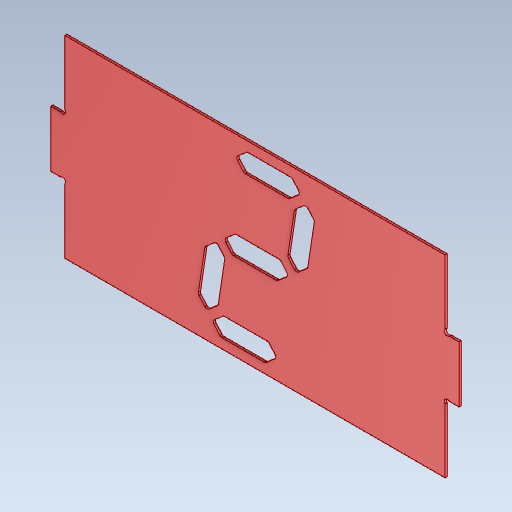
# Autodesk Inventor part: Cockpit_front_frame_cloth
Saved by Autodesk Inventor 2020 (Build 240168000, 168)
## iProperties
Part Number: Cockpit_front_frame_cloth
Material: PET プラスチック
Document SubType Name: Modeling
Designer: Masato Kubotera
Density: 1.541 g/cm^3
Appearance: 滑らか - 赤
Description: PP T0.75
Mass: 10.1319 g
Surface Area: 180.446 cm^2
Volume: 6.57488 cm^3
Author: Masato Kubotera
Autodesk Inventor part; units mm, degrees
ref_plane "YZ Plane" through (0, 0, 0) normal (1, 0, 0) x (0, 1, 0)
ref_plane "XZ Plane" through (0, 0, 0) normal (0, 1, 0) x (-1, 0, 0)
ref_plane "XY Plane" through (0, 0, 0) normal (0, 0, 1) x (1, 0, 0)
derived "Cockpit_front_frame.ipt"
sketch "スケッチ2" plane through (0, 0, 0) normal (0, 1, 0) x (-1, 0, 0)
  line L0 (-23.5, -22.5) -> (-28.5, -27.5)
  line L1 (-28.5, -27.5) -> (-28.5, -91)
  line L2 (-28.5, -91) -> (-23.5, -96)
  line L3 (-23.5, -96) -> (34.25, -96)
  line L4 (36.25, -98) -> (36.25, -131)
  line L5 (36.25, -131) -> (41.25, -136)
  line L6 (41.25, -136) -> (86.5, -136)
  line L7 (91.5, -131) -> (91.5, -20)
  line L8 (91.5, -20) -> (89, -17.5)
  line L9 (89, -17.5) -> (83.25, -17.5)
  line L10 (83.25, -17.5) -> (83.25, -21.0151)
  line L11 (81.7651, -22.5) -> (76.9849, -22.5)
  line L12 (75.5, -21.0151) -> (75.5, -17.5)
  line L13 (75.5, -17.5) -> (67.5, -17.5)
  line L14 (67.5, -17.5) -> (67.5, -21.0151)
  line L15 (66.0151, -22.5) -> (-23.5, -22.5)
  line L16 (-25.25, -25) -> (-20.25, -25) construction
  line L17 (-20.25, -25) -> (-20.25, -93.5) construction
  line L18 (-20.25, -93.5) -> (-25.25, -93.5) construction
  line L19 (-25.25, -93.5) -> (-25.25, -25) construction
  line L20 (-26, -25) -> (-25.25, -25) construction
  line L21 (-25.25, -93.5) -> (-26, -93.5) construction
  line L22 (-26, -93.5) -> (-26, -25) construction
  line L23 (-20.25, -93.5) -> (83.25, -93.5) construction
  line L24 (-20.25, -88.5) -> (83.25, -88.5) construction
  line L25 (83.25, -22.5) -> (83.25, -90.5) construction
  line L26 (83.25, -90.5) -> (88.25, -90.5) construction
  line L27 (88.25, -90.5) -> (88.25, -22.5) construction
  line L28 (83.25, -88.5) -> (83.25, -93.5) construction
  line L29 (83.25, -91) -> (88.25, -91) construction
  line L30 (88.25, -91) -> (88.25, -133.5) construction
  line L31 (83.25, -91) -> (83.25, -133.5) construction
  line L32 (83.25, -133.5) -> (88.25, -133.5) construction
  line L33 (38.75, -133.5) -> (38.75, -128.5) construction
  line L34 (38.75, -128.5) -> (38.75, -93.5) construction
  line L35 (43.75, -93.5) -> (43.75, -128.5) construction
  line L36 (38.75, -128.5) -> (43.75, -128.5) construction
  line L37 (41.25, -128.5) -> (41.25, -93.5) construction
  line L38 (38.75, -128.5) -> (82.1145, -128.5) construction
  line L39 (82.1145, -128.5) -> (82.1145, -133.5) construction
  line L40 (82.1145, -133.5) -> (38.75, -133.5) construction
  line L41 (38.75, -131) -> (82.1145, -131) construction
  line L42 (85.75, -91) -> (85.75, -133.5) construction
  circle A0 centre (85.75, -131) radius 2
  arc A1 (83.25, -128.5) -> (88.25, -128.5) centre (85.75, -131) ccw construction
  line L43 (83.25, -91) -> (-20.25, -91) construction
  line L44 (41.25, -111) -> (43.75, -111) construction
  line L45 (60.4322, -128.5) -> (60.4322, -131) construction
  line L46 (41.2, -115.5651) -> (41.2, -106.4349)
  line L47 (43.8, -107.05) -> (43.8, -114.95)
  line L48 (43.8, -117.05) -> (41.2, -104.95) construction
  line L49 (41.2, -117.05) -> (43.8, -104.95) construction
  line L50 (56.4822, -128.45) -> (64.3822, -128.45)
  line L51 (64.9973, -131.05) -> (55.8672, -131.05)
  line L52 (54.3822, -128.45) -> (66.4822, -131.05) construction
  line L53 (66.4822, -128.45) -> (54.3822, -131.05) construction
  line L54 (41.25, -105) -> (43.75, -105) construction
  line L55 (41.25, -117) -> (43.75, -117) construction
  arc A2 (42.6849, -104.95) -> (41.2, -106.4349) centre (41.9425, -105.6925) ccw
  arc A3 (43.8, -107.05) -> (43.8, -104.95) centre (43.8, -106) ccw
  arc A4 (41.2, -115.5651) -> (42.6849, -117.05) centre (41.9425, -116.3075) ccw
  arc A5 (43.8, -117.05) -> (43.8, -114.95) centre (43.8, -116) ccw
  line L56 (54.4322, -131) -> (54.4322, -128.5) construction
  line L57 (66.4322, -128.5) -> (66.4322, -131) construction
  arc A6 (54.3822, -129.5651) -> (55.8672, -131.05) centre (55.1247, -130.3075) ccw
  arc A7 (56.4822, -128.45) -> (54.3822, -128.45) centre (55.4322, -128.45) ccw
  arc A8 (64.9973, -131.05) -> (66.4822, -129.5651) centre (65.7398, -130.3075) ccw
  arc A9 (66.4822, -128.45) -> (64.3822, -128.45) centre (65.4322, -128.45) ccw
  line L58 (54.3822, -129.5651) -> (54.3822, -128.45)
  line L59 (66.4822, -128.45) -> (66.4822, -129.5651)
  line L60 (42.6849, -104.95) -> (43.8, -104.95)
  line L61 (43.8, -117.05) -> (42.6849, -117.05)
  circle A10 centre (48.4322, -131) radius 1.6
  line L62 (88.25, -22.5) -> (88.25, -17.5) construction
  line L63 (89, -17.5) -> (89, -90.5) construction
  line L64 (89, -90.5) -> (88.25, -90.5) construction
  line L65 (-13.5, -82.5) -> (-13.5, -61)
  arc A11 (-13.5, -82.5) -> (-11.5, -84.5) centre (-11.5, -82.5) ccw
  line L66 (45.5, -84.5) -> (-11.5, -84.5)
  arc A12 (45.5, -84.5) -> (47.5, -82.5) centre (45.5, -82.5) ccw
  line L67 (47.5, -61) -> (47.5, -82.5)
  arc A13 (47.5, -61) -> (45.5, -59) centre (45.5, -61) ccw
  line L68 (-11.5, -59) -> (45.5, -59)
  arc A14 (-11.5, -59) -> (-13.5, -61) centre (-11.5, -61) ccw
  line L69 (31.5, -88.5) -> (31.5, -91) construction
  line L70 (85.75, -22.5) -> (85.75, -90.5) construction
  circle A15 centre (85.75, -34) radius 1.6
  circle A16 centre (85.75, -34) radius 3
  circle A17 centre (85.75, -79) radius 1.6
  circle A18 centre (85.75, -79) radius 3
  line L71 (88.25, -22.5) -> (83.25, -22.5) construction
  arc A19 (88.25, -91) -> (83.25, -91) centre (85.75, -131) ccw construction
  circle A20 centre (48.4322, -131) radius 3
  circle A21 centre (41.25, -99) radius 1.6
  circle A22 centre (41.25, -99) radius 3
  line L72 (6.5, -88.5) -> (6.5, -91) construction
  line L73 (56.5, -88.5) -> (56.5, -91) construction
  line L74 (55.0651, -91.05) -> (7.9349, -91.05)
  line L75 (6.45, -89.5651) -> (6.45, -88.45)
  line L76 (8.55, -88.45) -> (54.45, -88.45)
  line L77 (56.55, -88.45) -> (56.55, -89.5651)
  line L78 (56.55, -91.05) -> (6.45, -88.45) construction
  line L79 (6.45, -91.05) -> (56.55, -88.45) construction
  arc A23 (8.55, -88.45) -> (6.45, -88.45) centre (7.5, -88.45) ccw
  arc A24 (6.45, -89.5651) -> (7.9349, -91.05) centre (7.1925, -90.3075) ccw
  arc A25 (56.55, -88.45) -> (54.45, -88.45) centre (55.5, -88.45) ccw
  arc A26 (55.0651, -91.05) -> (56.55, -89.5651) centre (55.8075, -90.3075) ccw
  line L80 (-20.25, -41) -> (83.25, -41) construction
  line L81 (83.25, -36) -> (-20.25, -36) construction
  line L82 (-20.25, -36) -> (-20.25, -41) construction
  line L83 (-20.25, -38.5) -> (83.25, -38.5) construction
  line L84 (31.5, -41) -> (31.5, -36) construction
  line L85 (55.0651, -35.95) -> (7.9349, -35.95)
  line L86 (7.9349, -41.05) -> (55.0651, -41.05)
  line L87 (56.55, -35.95) -> (6.45, -41.05) construction
  line L88 (6.45, -35.95) -> (55.5877, -40.952) construction
  arc A27 (7.9349, -35.95) -> (6.45, -37.4349) centre (7.1925, -36.6925) ccw
  arc A28 (6.45, -39.5651) -> (7.9349, -41.05) centre (7.1925, -40.3075) ccw
  arc A29 (56.55, -37.4349) -> (55.0651, -35.95) centre (55.8075, -36.6925) ccw
  arc A30 (55.0651, -41.05) -> (56.55, -39.5651) centre (55.8075, -40.3075) ccw
  line L89 (6.5, -41) -> (6.5, -36) construction
  line L90 (56.5, -36) -> (56.5, -41) construction
  line L91 (6.45, -37.4349) -> (6.45, -39.5651)
  line L92 (56.55, -39.5651) -> (56.55, -37.4349)
  circle A31 centre (-1, -38.5) radius 1.6
  circle A32 centre (-1, -38.5) radius 3
  circle A33 centre (64, -38.5) radius 1.6
  circle A34 centre (64, -38.5) radius 3
  line L93 (-25.25, -49.25) -> (-26, -49.25) construction
  line L94 (-25.25, -69.25) -> (-26, -69.25) construction
  line L95 (-26, -59.25) -> (-25.25, -59.25) construction
  line L96 (-22.75, -25) -> (-22.75, -93.5) construction
  arc A35 (66.0151, -22.5) -> (67.5, -21.0151) centre (66.7575, -21.7575) ccw
  arc A36 (75.5, -21.0151) -> (76.9849, -22.5) centre (76.2425, -21.7575) ccw
  line L97 (59.75, -22.5) -> (59.75, -32.5) construction
  line L98 (59.75, -32.5) -> (83.25, -32.5) construction
  line L99 (83.25, -32.5) -> (83.25, -22.5) construction
  line L100 (71.5, -17.5) -> (71.5, -32.5) construction
  line L101 (63.5, -22.5) -> (63.5, -17.5) construction
  line L102 (79.5, -22.5) -> (79.5, -17.5) construction
  circle A37 centre (-22.75, -31.75) radius 1.6
  circle A38 centre (-22.75, -31.75) radius 3
  circle A39 centre (-22.75, -86.75) radius 1.6
  circle A40 centre (-22.75, -86.75) radius 3
  line L103 (67.5, -22.5) -> (75.5, -22.5)
  line L104 (88.25, -17.5) -> (52.5, -17.5) construction
  line L105 (52.5, -17.5) -> (52.5, -22.5) construction
  circle A41 centre (85.75, -98.5) radius 1.475
  circle A42 centre (85.75, -103.5) radius 1.475
  circle A43 centre (85.75, -108.5) radius 1.475
  line L106 (48.25, -93.5) -> (78.75, -93.5)
  line L107 (80.75, -95.5) -> (80.75, -124)
  line L108 (78.75, -126) -> (48.25, -126)
  line L109 (46.25, -124) -> (46.25, -95.5)
  arc A44 (48.25, -93.5) -> (46.25, -95.5) centre (48.25, -95.5) ccw
  arc A45 (46.25, -124) -> (48.25, -126) centre (48.25, -124) ccw
  arc A46 (78.75, -126) -> (80.75, -124) centre (78.75, -124) ccw
  arc A47 (80.75, -95.5) -> (78.75, -93.5) centre (78.75, -95.5) ccw
  arc A48 (36.25, -98) -> (34.25, -96) centre (34.25, -98) ccw
  circle A49 centre (-13.5, -55) radius 1.75
  circle A50 centre (-13.5, -55) radius 2
  line L110 (77.85, -78.65) -> (68.65, -78.65) construction
  line L111 (68.65, -78.65) -> (68.65, -64.85) construction
  line L112 (68.65, -64.85) -> (77.85, -64.85) construction
  line L113 (77.85, -64.85) -> (77.85, -78.65) construction
  line L114 (77.85, -78.65) -> (68.65, -64.85) construction
  line L115 (68.65, -78.65) -> (77.85, -64.85) construction
  line L116 (67.95, -64.2) -> (78.55, -64.2) construction
  line L117 (78.55, -64.2) -> (78.55, -79.3) construction
  line L118 (78.55, -79.3) -> (67.95, -79.3) construction
  line L119 (67.95, -79.3) -> (67.95, -64.2) construction
  line L120 (67.95, -64.2) -> (78.55, -79.3) construction
  line L121 (78.55, -64.2) -> (67.95, -79.3) construction
  line L122 (69.3849, -64.15) -> (77.1151, -64.15)
  line L123 (78.6, -65.6349) -> (78.6, -77.8651)
  line L124 (78.6, -79.35) -> (67.9, -64.15) construction
  line L125 (67.9, -79.35) -> (78.6, -64.15) construction
  line L126 (77.9, -78.7) -> (68.6, -64.8) construction
  line L127 (68.6, -78.7) -> (77.9, -64.8) construction
  arc A51 (69.3849, -64.15) -> (67.9, -65.6349) centre (68.6425, -64.8925) ccw
  arc A52 (70.0849, -64.8) -> (68.6, -66.2849) centre (69.3425, -65.5425) ccw
  line L128 (67.9, -71.75) -> (78.6, -71.75) construction
  line L129 (73.25, -64.15) -> (73.25, -78.7063) construction
  arc A53 (78.6, -65.6349) -> (77.1151, -64.15) centre (77.8575, -64.8925) ccw
  arc A54 (77.9, -66.2849) -> (76.4151, -64.8) centre (77.1575, -65.5425) ccw
  arc A55 (67.9, -77.8651) -> (69.3849, -79.35) centre (68.6425, -78.6075) ccw
  arc A56 (68.6, -77.2151) -> (70.0849, -78.7) centre (69.3425, -77.9575) ccw
  arc A57 (77.1151, -79.35) -> (78.6, -77.8651) centre (77.8575, -78.6075) ccw
  arc A58 (76.4151, -78.7) -> (77.9, -77.2151) centre (77.1575, -77.9575) ccw
  line L130 (70.0849, -64.8) -> (76.4151, -64.8)
  line L131 (77.9, -66.2849) -> (77.9, -77.2151)
  line L132 (67.9, -77.8651) -> (67.9, -65.6349)
  line L133 (68.6, -77.2151) -> (68.6, -66.2849)
  line L134 (76.4151, -78.7) -> (70.0849, -78.7)
  line L135 (77.1151, -79.35) -> (69.3849, -79.35)
  line L136 (-13.5, -71.75) -> (47.5, -71.75) construction
  line L137 (85.75, -56.5) -> (88.25, -56.5) construction
  line L138 (89, -54) -> (88.25, -54) construction
  line L139 (85.7, -69.45) -> (85.7, -43.55)
  line L140 (88.2835, -71.3588) -> (85.7, -41.45) construction
  line L141 (85.7, -71.55) -> (88.3, -41.45) construction
  arc A59 (85.7, -41.45) -> (85.7, -43.55) centre (85.7, -42.5) ccw
  arc A60 (88.3, -42.9349) -> (86.8151, -41.45) centre (87.5575, -42.1925) ccw
  arc A61 (85.7, -69.45) -> (85.7, -71.55) centre (85.7, -70.5) ccw
  arc A62 (86.8151, -71.55) -> (88.3, -70.0651) centre (87.5575, -70.8075) ccw
  line L142 (85.75, -41.5) -> (88.25, -41.5) construction
  line L143 (85.75, -71.5) -> (88.25, -71.5) construction
  arc A63 (89.25, -47.1801) -> (88.3, -46.1348) centre (88.2, -47.1801) ccw
  line L144 (89.25, -47.1801) -> (89.25, -65.8199)
  line L145 (88.25, -46.5) -> (89, -46.5) construction
  line L146 (88.25, -66.5) -> (89, -66.5) construction
  arc A64 (88.3, -66.8652) -> (89.25, -65.8199) centre (88.2, -65.8199) ccw
  line L147 (88.3, -42.9349) -> (88.3, -46.1348)
  line L148 (88.3, -66.8652) -> (88.3, -70.0651)
  line L149 (86.8151, -71.55) -> (85.7, -71.55)
  line L150 (85.7, -41.45) -> (86.8151, -41.45)
  line L151 (86.5, -136) -> (91.5, -131)
  arc A65 (81.7651, -22.5) -> (83.25, -21.0151) centre (82.5075, -21.7575) ccw
  circle A66 centre (85.75, -93.5) radius 2
  circle A67 centre (85.75, -93.5) radius 4 construction
  arc A68 (-24.15, -49.25) -> (-26.25, -49.25) centre (-25.2, -49.25) ccw
  line L152 (-26, -49.25) -> (-26.25, -49.25) construction
  line L153 (-26.25, -49.25) -> (-26.25, -69.25)
  line L154 (-24.15, -49.25) -> (-24.15, -69.25)
  arc A69 (-26.25, -69.25) -> (-24.15, -69.25) centre (-25.2, -69.25) ccw
  point P0 (0, 0)
  point P1 (-25.7227, -96)
  point P2 (-23.5, -22.5)
  point P3 (42.5, -111)
  point P4 (60.4322, -129.75)
  point P5 (31.5, -89.75)
  point P6 (31.5, -38.5)
  point P7 (6.45, -41.05)
  point P8 (52.5, -22)
  point P9 (73.25, -71.75)
  point P10 (73.25, -71.75)
  point P11 (87, -56.5)
  dimension "d4" = 0.75
  measures "d4" distance of L20.start L20.end
sketch "スケッチ3" plane through (25.25, 0, 0) normal (1, 0, 0) x (0, 1, 0)
  line L0 (-135, -25) -> (0, -25)
  line L1 (0, -93.5) -> (-135, -93.5)
  line L2 (0, -25) -> (0, -93.5)
  line L3 (0, -75.7349) -> (0, -93.5)
  line L4 (-67.5, -25) -> (-67.5, -93.5) construction
  line L5 (-135, -25) -> (-135, -93.5)
  line L6 (-7, -30) -> (-128, -30)
  line L7 (-130, -32) -> (-130, -34)
  line L8 (-128, -36) -> (-7, -36)
  line L9 (-5, -34) -> (-5, -32)
  line L10 (-5, -30) -> (-130, -36) construction
  line L11 (-130, -30) -> (-5, -36) construction
  line L12 (-7, -88.5) -> (-128, -88.5)
  line L13 (-130, -86.5) -> (-130, -43)
  line L14 (-128, -41) -> (-7, -41)
  line L15 (-5, -43) -> (-5, -86.5)
  line L16 (-5, -88.5) -> (-130, -41) construction
  line L17 (-130, -88.5) -> (-5, -41) construction
  arc A0 (-128, -30) -> (-130, -32) centre (-128, -32) ccw
  arc A1 (-130, -34) -> (-128, -36) centre (-128, -34) ccw
  arc A2 (-7, -36) -> (-5, -34) centre (-7, -34) ccw
  arc A3 (-5, -32) -> (-7, -30) centre (-7, -32) ccw
  arc A4 (-5, -43) -> (-7, -41) centre (-7, -43) ccw
  arc A5 (-128, -41) -> (-130, -43) centre (-128, -43) ccw
  arc A6 (-130, -86.5) -> (-128, -88.5) centre (-128, -86.5) ccw
  arc A7 (-7, -88.5) -> (-5, -86.5) centre (-7, -86.5) ccw
  point P0 (0, 0)
  point P1 (-135, -93.5)
  point P2 (-135, -25)
  point P3 (-67.5, -33)
  point P4 (-67.5, -64.75)
  point P5 (0, -36)
  point P6 (0, -36)
  point P7 (0, -36)
  point P8 (0, -41)
  point P9 (0, -41)
  point P10 (0, -41)
ref_plane "作業平面1" through (25.25, -135, -25) normal (-1, 0, 0) x (0, 1, 0)
sketch "スケッチ4" plane through (25.25, -135, -25) normal (-1, 0, 0) x (0, 1, 0)
  arc A0 (136.4849, 24.25) -> (135, 22.7651) centre (135.7425, 23.5075) ccw
  line L0 (136.4849, 24.25) -> (140, 24.25)
  line L1 (140, 24.25) -> (140, 44.25)
  line L2 (67.5, 0) -> (67.5, 68.5) construction
  line L3 (0, 0) -> (135, 0) projected
  line L4 (135, 68.5) -> (0, 68.5) projected
  arc A1 (135, 45.7349) -> (136.4849, 44.25) centre (135.7425, 44.9925) ccw
  line L5 (136.4849, 44.25) -> (140, 44.25)
  line L6 (135, 22.7651) -> (135, 0)
  line L7 (135, 45.7349) -> (135, 68.5)
  arc A2 (0, 22.7651) -> (-1.4849, 24.25) centre (-0.7425, 23.5075) ccw
  line L8 (-1.4849, 24.25) -> (-5, 24.25)
  line L9 (-1.4849, 44.25) -> (-5, 44.25)
  arc A3 (-1.4849, 44.25) -> (0, 45.7349) centre (-0.7425, 44.9925) ccw
  line L10 (0, 22.7651) -> (0, 0)
  line L11 (0, 45.7349) -> (0, 68.5)
  line L12 (-5, 24.25) -> (-5, 44.25)
  line L13 (51.1141, 58.6095) -> (54.1517, 56.0021)
  line L14 (53.0682, 60.8859) -> (56.1057, 58.2784)
  line L15 (55.0145, 64.6885) -> (52.9607, 62.296)
  line L16 (49.704, 58.5021) -> (47.6502, 56.1095)
  line L17 (55.7733, 65.0372) -> (70.8617, 65.0372)
  line L18 (72.6043, 58.3859) -> (74.658, 60.7784)
  line L19 (71.513, 64.796) -> (74.5506, 62.1885)
  line L20 (56.7571, 58.0372) -> (71.8455, 58.0372)
  line L21 (54.4888, 55.3948) -> (56.7748, 40.4805)
  line L22 (56.5452, 39.6777) -> (54.4914, 37.2851)
  line L23 (53.0813, 37.1777) -> (50.0437, 39.7851)
  line L24 (47.4206, 55.3066) -> (49.7066, 40.3924)
  line L25 (50.3553, 59.2608) -> (53.84, 36.5264) construction
  line L26 (75.3094, 61.5372) -> (52.3094, 61.5372) construction
  arc A4 (51.1141, 58.6095) -> (49.704, 58.5021) centre (50.4628, 57.8507) ccw
  arc A5 (54.4888, 55.3948) -> (54.1517, 56.0021) centre (53.5003, 55.2433) ccw
  arc A6 (56.5452, 39.6777) -> (56.7748, 40.4805) centre (55.7864, 40.329) ccw
  arc A7 (53.0813, 37.1777) -> (54.4914, 37.2851) centre (53.7326, 37.9365) ccw
  arc A8 (49.7066, 40.3924) -> (50.0437, 39.7851) centre (50.695, 40.5439) ccw
  arc A9 (47.6502, 56.1095) -> (47.4206, 55.3066) centre (48.409, 55.4582) ccw
  arc A10 (71.8455, 58.0372) -> (72.6043, 58.3859) centre (71.8455, 59.0372) ccw
  arc A11 (74.658, 60.7784) -> (74.5506, 62.1885) centre (73.8992, 61.4298) ccw
  arc A12 (71.513, 64.796) -> (70.8617, 65.0372) centre (70.8617, 64.0372) ccw
  arc A13 (55.7733, 65.0372) -> (55.0145, 64.6885) centre (55.7733, 64.0372) ccw
  arc A14 (52.9607, 62.296) -> (53.0682, 60.8859) centre (53.7195, 61.6446) ccw
  arc A15 (56.1057, 58.2784) -> (56.7571, 58.0372) centre (56.7571, 59.0372) ccw
  line L27 (78.72, 58.6095) -> (81.7576, 56.0021)
  line L28 (77.3099, 58.5021) -> (75.2561, 56.1095)
  arc A16 (78.72, 58.6095) -> (77.3099, 58.5021) centre (78.0687, 57.8507) ccw
  line L29 (75.0264, 55.3066) -> (77.3125, 40.3924)
  arc A17 (75.2561, 56.1095) -> (75.0264, 55.3066) centre (76.0149, 55.4582) ccw
  arc A18 (82.0947, 55.3948) -> (81.7576, 56.0021) centre (81.1062, 55.2433) ccw
  line L30 (82.0947, 55.3948) -> (84.3807, 40.4805)
  arc A19 (84.151, 39.6777) -> (84.3807, 40.4805) centre (83.3922, 40.329) ccw
  line L31 (84.151, 39.6777) -> (82.0973, 37.2851)
  arc A20 (80.6871, 37.1777) -> (82.0973, 37.2851) centre (81.3385, 37.9365) ccw
  line L32 (80.6871, 37.1777) -> (77.6496, 39.7851)
  arc A21 (77.3125, 40.3924) -> (77.6496, 39.7851) centre (78.3009, 40.5439) ccw
  line L33 (55.2967, 31.3223) -> (58.3342, 28.7149)
  line L34 (53.8865, 31.2149) -> (51.8328, 28.8223)
  arc A22 (55.2967, 31.3223) -> (53.8865, 31.2149) centre (54.6453, 30.5635) ccw
  line L35 (51.6031, 28.0195) -> (53.8891, 13.1052)
  arc A23 (51.8328, 28.8223) -> (51.6031, 28.0195) centre (52.5915, 28.171) ccw
  arc A24 (58.6713, 28.1076) -> (58.3342, 28.7149) centre (57.6829, 27.9561) ccw
  line L36 (58.6713, 28.1076) -> (60.9573, 13.1934)
  arc A25 (60.7277, 12.3905) -> (60.9573, 13.1934) centre (59.9689, 13.0418) ccw
  line L37 (60.7277, 12.3905) -> (58.6739, 9.9979)
  arc A26 (57.2638, 9.8905) -> (58.6739, 9.9979) centre (57.9151, 10.6493) ccw
  line L38 (57.2638, 9.8905) -> (54.2262, 12.4979)
  arc A27 (53.8891, 13.1052) -> (54.2262, 12.4979) centre (54.8776, 13.2567) ccw
  line L39 (82.9025, 31.3223) -> (85.9401, 28.7149)
  line L40 (81.4924, 31.2149) -> (79.4386, 28.8223)
  arc A28 (82.9025, 31.3223) -> (81.4924, 31.2149) centre (82.2512, 30.5635) ccw
  line L41 (79.209, 28.0195) -> (81.495, 13.1052)
  arc A29 (79.4386, 28.8223) -> (79.209, 28.0195) centre (80.1974, 28.171) ccw
  arc A30 (86.2772, 28.1076) -> (85.9401, 28.7149) centre (85.2887, 27.9561) ccw
  line L42 (86.2772, 28.1076) -> (88.5632, 13.1934)
  arc A31 (88.3336, 12.3905) -> (88.5632, 13.1934) centre (87.5748, 13.0418) ccw
  line L43 (88.3336, 12.3905) -> (86.2798, 9.9979)
  arc A32 (84.8697, 9.8905) -> (86.2798, 9.9979) centre (85.521, 10.6493) ccw
  line L44 (84.8697, 9.8905) -> (81.8321, 12.4979)
  arc A33 (81.495, 13.1052) -> (81.8321, 12.4979) centre (82.4834, 13.2567) ccw
  line L45 (59.9558, 37.75) -> (75.0442, 37.75)
  arc A34 (59.9558, 37.75) -> (59.197, 37.4013) centre (59.9558, 36.75) ccw
  line L46 (59.197, 37.4013) -> (57.1432, 35.0088)
  arc A35 (57.1432, 35.0088) -> (57.2507, 33.5987) centre (57.902, 34.3574) ccw
  line L47 (57.2507, 33.5987) -> (60.2882, 30.9912)
  arc A36 (60.2882, 30.9912) -> (60.9396, 30.75) centre (60.9396, 31.75) ccw
  line L48 (60.9396, 30.75) -> (76.028, 30.75)
  arc A37 (76.028, 30.75) -> (76.7868, 31.0987) centre (76.028, 31.75) ccw
  line L49 (76.7868, 31.0987) -> (78.8406, 33.4912)
  arc A38 (78.8406, 33.4912) -> (78.7331, 34.9013) centre (78.0818, 34.1426) ccw
  line L50 (75.6955, 37.5088) -> (78.7331, 34.9013)
  arc A39 (75.6955, 37.5088) -> (75.0442, 37.75) centre (75.0442, 36.75) ccw
  line L51 (64.1383, 10.4628) -> (79.2267, 10.4628)
  arc A40 (64.1383, 10.4628) -> (63.3795, 10.1141) centre (64.1383, 9.4628) ccw
  line L52 (63.3795, 10.1141) -> (61.3258, 7.7216)
  arc A41 (61.3258, 7.7216) -> (61.4332, 6.3115) centre (62.0845, 7.0702) ccw
  line L53 (61.4332, 6.3115) -> (64.4708, 3.704)
  arc A42 (64.4708, 3.704) -> (65.1221, 3.4628) centre (65.1221, 4.4628) ccw
  line L54 (65.1221, 3.4628) -> (80.2105, 3.4628)
  arc A43 (80.2105, 3.4628) -> (80.9693, 3.8115) centre (80.2105, 4.4628) ccw
  line L55 (80.9693, 3.8115) -> (83.0231, 6.204)
  arc A44 (83.0231, 6.204) -> (82.9156, 7.6141) centre (82.2643, 6.8554) ccw
  line L56 (79.8781, 10.2216) -> (82.9156, 7.6141)
  arc A45 (79.8781, 10.2216) -> (79.2267, 10.4628) centre (79.2267, 9.4628) ccw
  line L57 (67.5, 37.75) -> (68.4838, 30.75) construction
  line L58 (-5, 34.25) -> (140, 34.25) construction
  point P0 (135, -25)
  point P1 (135, 24.25)
  point P2 (135, 24.25)
  point P3 (135, 24.25)
  point P4 (135, 24.25)
  point P5 (47.3509, 55.7608)
  point P6 (54.4327, 55.7608)
  point P7 (56.3867, 58.0372)
  point P8 (55.3138, 65.0372)
  point P9 (71.232, 65.0372)
  point P10 (72.305, 58.0372)
  point P11 (56.8444, 40.0264)
  point P12 (49.7627, 40.0264)
  point P13 (77.9612, 59.2608)
  point P14 (82.0386, 55.7608)
  point P15 (74.9568, 55.7608)
  point P16 (77.3686, 40.0264)
  point P17 (84.4503, 40.0264)
  point P18 (81.4459, 36.5264)
  point P19 (54.5379, 31.9736)
  point P20 (58.6152, 28.4736)
  point P21 (51.5335, 28.4736)
  point P22 (53.9452, 12.7392)
  point P23 (61.027, 12.7392)
  point P24 (58.0226, 9.2392)
  point P25 (82.1437, 31.9736)
  point P26 (86.2211, 28.4736)
  point P27 (79.1393, 28.4736)
  point P28 (81.5511, 12.7392)
  point P29 (88.6328, 12.7392)
  point P30 (85.6284, 9.2392)
  point P31 (75.4145, 37.75)
  point P32 (59.4963, 37.75)
  point P33 (56.4919, 34.25)
  point P34 (60.5692, 30.75)
  point P35 (76.4875, 30.75)
  point P36 (79.4919, 34.25)
  point P37 (79.5971, 10.4628)
  point P38 (63.6788, 10.4628)
  point P39 (60.6744, 6.9628)
  point P40 (64.7518, 3.4628)
  point P41 (80.67, 3.4628)
  point P42 (83.6744, 6.9628)
  point P43 (135, 44.25)
  point P44 (135, 44.25)
  point P45 (135, 44.25)
  point P46 (135, 44.25)
  point P47 (67.9919, 34.25)
  dimension "d1" = 1.05
  dimension "d13" = 3
  dimension "d14" = 7
  dimension "d15" = 7
  dimension "d16" = 23
  dimension "d17" = 23
  dimension "d18" = 1
  dimension "d19" = 1
  dimension "d20" = 27.6059
  dimension "d21" = 27.6059
  dimension "d22" = 27.6059
  dimension "d26" = 5
  dimension "d27" = 8
  constraints: 112 end point, 94 point on circle, 92 point on line, 46 centre point, 24 tangent, 10 equal radius, 8 symmetric about line, 6 collinear, 6 parallel, 5 midpoint, 3 perpendicular, 2 horizontal, 1 vertical, 187 other
  measures "d1" radius of A0
  measures "d13" distance between parallel lines of L13 L14
  measures "d14" distance between parallel lines of L20 L17
  measures "d15" distance between parallel lines of L21 L24
  measures "d16" distance of L26.start L26.end
  measures "d17" distance of L25.start L25.end
  measures "d18" radius of A4
  measures "d19" radius of A10
  measures "d20" distance of L13.start L27.start
  measures "d21" distance of L13.start L33.start
  measures "d22" distance of L17.start L45.start
  measures "d26" distance between parallel lines of L6 L1
  measures "d27" angle of L57 L2
extrude "押し出し1" add sketch "スケッチ4" against normal blind 0.75 contours A0 L6 L3 L10 A2 L8 L12 L9 A3 L11 L4 L7 A1 L5 L1 L0 | L27 A18 L30 A19 L31 A20 L32 A21 L29 A17 L28 A16 | L33 A24 L36 A25 L37 A26 L38 A27 L35 A23 L34 A22
equation "\"d15\" = d14"
equation "\"d17\" = d16"
equation "\"d2\" = d4"
